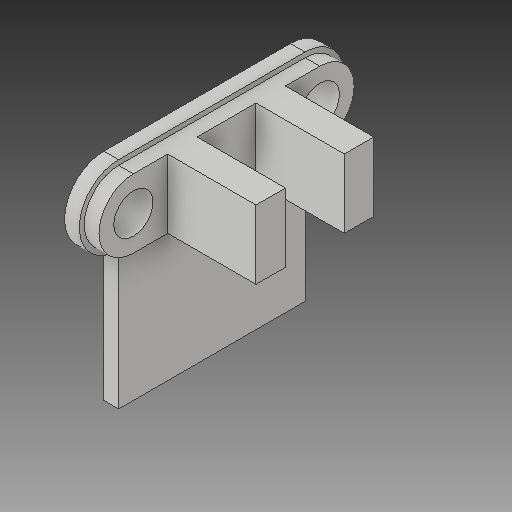
# Autodesk Inventor part: HC020K
Saved by Autodesk Inventor 2019 (Build 230136000, 136)
## iProperties
Created: 2022-09-15
Part Number: HC020K
Material: Generic
Document SubType Name: Modeling
Designer: ThinkPad
Density: 2.37675 g/cm^3
Appearance: Default
Mass: 3 g
Surface Area: 15.4835 cm^2
Volume: 1.26223 cm^3
Author: ThinkPad
Autodesk Inventor part; units mm, degrees
ref_plane "YZ Plane" through (0, 0, 0) normal (1, 0, 0) x (0, 1, 0)
ref_plane "XZ Plane" through (0, 0, 0) normal (0, 1, 0) x (-1, 0, 0)
ref_plane "XY Plane" through (0, 0, 0) normal (0, 0, 1) x (1, 0, 0)
sketch "Sketch1" plane through (0, 0, 0) normal (1, 0, 0) x (0, 1, 0)
  line L0 (-14.1111, 2.4111) -> (-14.1111, -16.5889)
  line L1 (7.8889, -16.5889) -> (7.8889, 2.4111)
  arc A0 (7.8889, 2.4111) -> (-0.1111, 2.4111) centre (3.8889, 2.4111) ccw
  arc A1 (-0.1111, -16.5889) -> (7.8889, -16.5889) centre (3.8889, -16.5889) ccw
  line L2 (-0.1111, 2.4111) -> (-14.1111, 2.4111)
  line L3 (-0.1111, -16.5889) -> (-14.1111, -16.5889)
  line L4 (7.3889, -10.0889) -> (0.3889, -10.0889)
  line L5 (7.3889, -13.0889) -> (0.3889, -13.0889)
  line L6 (7.3889, -4.0889) -> (0.3889, -4.0889)
  line L7 (7.3889, -1.0889) -> (0.3889, -1.0889)
  line L8 (7.3889, 2.4111) -> (7.3889, -16.5889)
  arc A2 (0.3889, -16.5889) -> (7.3889, -16.5889) centre (3.8889, -16.5889) ccw
  arc A3 (7.3889, 2.4111) -> (0.3889, 2.4111) centre (3.8889, 2.4111) ccw
  line L9 (0.3889, 2.4111) -> (0.3889, -16.5889)
  circle A4 centre (3.8889, 2.4111) radius 2
  circle A5 centre (3.8889, -16.5889) radius 2
  point P0 (0, 0)
  dimension "d5" = 0.5
  dimension "d6" = 4
  dimension "d7" = 4
  constraints: 20 end point, 8 point on circle, 8 point on line, 6 centre point, 2 coincident, 2 perpendicular, 2 tangent, 1 parallel, 1 vertical
  measures "d5" distance between parallel lines of L1 L8
  measures "d6" diameter of A4
  measures "d7" diameter of A5
extrude "Extrusion1" add sketch "Sketch1" along normal blind 1.5 contours L2 A0 L1 A1 L3 L0 | L8 L5 L9 L4 | L4 L9 L6 L8 | L6 L9 L7 L8 | L8 A2 L9 L5 | L7 L9 A3 L8
extrude "Extrusion2" add sketch "Sketch1" along normal blind 3 contours L8 L5 L9 L4 | L4 L9 L6 L8 | L6 L9 L7 L8 | L8 A2 L9 L5 | L7 L9 A3 L8
extrude "Extrusion3" add sketch "Sketch1" along normal blind 12 contours L8 L5 L9 L4 | L6 L9 L7 L8
body "Solid1"
